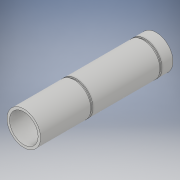
# Autodesk Inventor part: труба
Saved by Autodesk Inventor 2019.1 (Build 231200000, 200)
## iProperties
Created: 2018-08-23
Part Number: труба
Material: Типовые
Document SubType Name: Modeling
Designer: olege
Density: 1 g/cm^3
Appearance: По умолчанию
Author: olege
Autodesk Inventor part; units mm, degrees
ref_plane "YZ Plane" through (0, 0, 0) normal (1, 0, 0) x (0, 1, 0)
sketch "Эскиз1" plane through (0, 0, 0) normal (0, 0, 1) x (1, 0, 0)
  circle A0 centre (0, 0) radius 10
  circle A1 centre (0, 0) radius 8.5
  dimension "d1" = 20
  dimension "d2" = 17
  constraints: 2 centre point, 2 coincident
  measures "d1" diameter of A0
  measures "d2" diameter of A1
extrude "Выдавливание1" add sketch "Эскиз1" along normal blind 74
ref_plane "РабПлоскость1" through (0, 0, 33) normal (0, 0, -1) x (-1, 0, 0)
ref_plane "РабПлоскость2" through (0, 0, 40) normal (0, 0, 1) x (1, 0, 0)
sketch "Эскиз3" plane through (0, 0, 40) normal (0, 0, 1) x (1, 0, 0)
  circle A0 centre (0, 0) radius 8.5 projected
  circle A1 centre (0, 0) radius 9.25
  circle A2 centre (0, 0) radius 11
  dimension "d9" = 18.5
  dimension "d10" = 22
  constraints: 2 centre point, 2 coincident
  measures "d9" diameter of A1
  measures "d10" diameter of A2
extrude "Выдавливание3" cut sketch "Эскиз3" along normal blind 1.2 contours A2
ref_plane "РабПлоскость4" through (0, 0, 0) normal (0, 0, -1) x (-1, 0, 0)
ref_plane "РабПлоскость3" through (0, 0, 7) normal (0, 0, -1) x (-1, 0, 0)
sketch "Эскиз6" plane through (0, 0, 0) normal (0, 0, -1) x (-1, 0, 0)
  circle A0 centre (0, 0) radius 8.5 projected
  circle A1 centre (0, 0) radius 10 projected
extrude "Выдавливание6" add sketch "Эскиз6" along normal blind 15
sketch "Эскиз7" plane through (0, 0, 0) normal (0, 0, -1) x (-1, 0, 0)
  circle A0 centre (0, 0) radius 9.25
  circle A1 centre (0, 0) radius 11
  dimension "d25" = 18.5
  dimension "d26" = 22
  constraints: 2 centre point, 2 coincident
  measures "d25" diameter of A0
  measures "d26" diameter of A1
extrude "Выдавливание7" cut sketch "Эскиз7" along normal blind 1.2
sketch "Эскиз8" plane through (0, 0, 74) normal (0, 0, 1) x (1, 0, 0)
  circle A0 centre (0, 0) radius 19.934
  constraints: 1 centre point, 1 coincident
extrude "Выдавливание8" cut sketch "Эскиз8" against normal blind 2.8
sketch "Эскиз9" plane through (0, 0, -15) normal (0, 0, -1) x (-1, 0, 0)
  circle A0 centre (0, 0) radius 19.6449
  dimension "d33" = 39.2898
  constraints: 1 centre point, 1 coincident
  measures "d33" diameter of A0
extrude "Выдавливание9" cut sketch "Эскиз9" against normal blind 7.2
